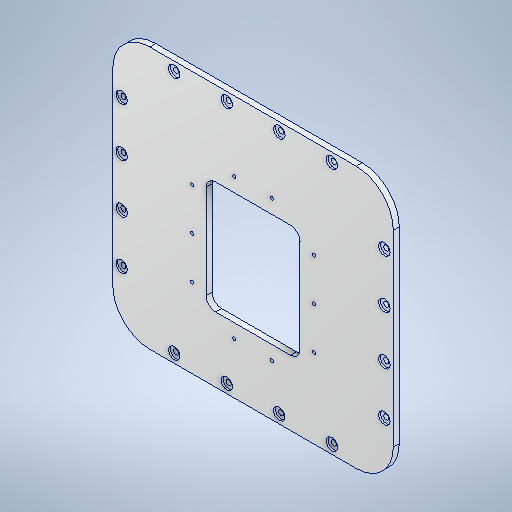
# Autodesk Inventor part: Reducer Plate
Saved by Autodesk Inventor 2025.2 (Build 292293000, 293)
## iProperties
Created: 2020-10-16
Part Number: Reducer Plate
Material: Aluminum 6061
Document SubType Name: Modeling
Designer: stabl
Density: 2.7 g/cm^3
Appearance: Aluminum - Flat
Author: stabl
Autodesk Inventor part; units mm, degrees
ref_plane "YZ Plane" through (0, 0, 0) normal (1, 0, 0) x (0, 1, 0)
ref_plane "XZ Plane" through (0, 0, 0) normal (0, 1, 0) x (-1, 0, 0)
ref_plane "Work Plane2" through (0, 0, 0) normal (0, 0, 1) x (1, 0, 0)
sketch "Sketch1" plane through (0, 0, 0) normal (0, 0, 1) x (1, 0, 0)
  line L0 (180, 126) -> (180, 200) projected
  arc A0 (180, 200) -> (175, 205) centre (175, 200) ccw projected
  line L1 (175, 205) -> (-174, 205) projected
  line L2 (-174, -368) -> (-174, 205) projected
  line L3 (-156, -368) -> (-174, -368) projected
  arc A1 (-153, -371) -> (-156, -368) centre (-156, -371) ccw projected
  line L4 (-153, -403) -> (-153, -371) projected
  arc A2 (-156, -406) -> (-153, -403) centre (-156, -403) ccw projected
  line L5 (-180, -406) -> (-156, -406) projected
  line L6 (-180, -406) -> (-180, -480) projected
  arc A3 (-180, -480) -> (-175, -485) centre (-175, -480) ccw projected
  line L7 (-175, -485) -> (174, -485) projected
  line L8 (174, 88) -> (174, -485) projected
  line L9 (156, 88) -> (174, 88) projected
  arc A4 (153, 91) -> (156, 88) centre (156, 91) ccw projected
  line L10 (153, 123) -> (153, 91) projected
  arc A5 (156, 126) -> (153, 123) centre (156, 123) ccw projected
  line L11 (180, 126) -> (156, 126) projected
  circle A6 centre (0, 0) radius 135 projected
  circle A7 centre (82.55, 185) radius 3 projected
  circle A8 centre (-82.55, 185) radius 3 projected
  circle A9 centre (82.55, -460) radius 3 projected
  circle A10 centre (-82.55, -460) radius 3 projected
  line L12 (-149.5, -195) -> (-149.5, -395)
  arc A11 (-149.5, -395) -> (-110, -434.5) centre (-110, -395) ccw
  line L13 (-110, -434.5) -> (110, -434.5)
  arc A12 (110, -434.5) -> (149.5, -395) centre (110, -395) ccw
  line L14 (149.5, -395) -> (149.5, -195)
  arc A13 (149.5, -195) -> (110, -155.5) centre (110, -195) ccw
  line L15 (110, -155.5) -> (-110, -155.5)
  arc A14 (-110, -155.5) -> (-149.5, -195) centre (-110, -195) ccw
  line L16 (40, -245) -> (-40, -245)
  line L17 (-50, -255) -> (-50, -355)
  line L18 (-40, -365) -> (40, -365)
  line L19 (50, -355) -> (50, -255)
  arc A15 (-40, -245) -> (-50, -255) centre (-40, -255) ccw
  arc A16 (50, -255) -> (40, -245) centre (40, -255) ccw
  arc A17 (40, -365) -> (50, -355) centre (40, -355) ccw
  arc A18 (-50, -355) -> (-40, -365) centre (-40, -355) ccw
  point P0 (115, -175)
  point P1 (-50, -365)
  point P2 (-50, -245)
  point P3 (50, -365)
  dimension "d1" = 100
  dimension "d2" = 120
  dimension "d3" = 10
  constraints: 16 end point, 16 point on circle, 8 centre point, 8 tangent, 6 point on line, 3 equal radius, 2 horizontal, 2 parallel, 1 perpendicular
  measures "d1" distance of point (50, -365) point (-50, -365)
  measures "d2" distance of point (-50, -365) point (-50, -245)
  measures "d3" radius of A15
extrude "Extrusion1" add sketch "Sketch1" along normal blind 6.35 contours A14 L15 A13 L14 A12 L13 A11 L12
sketch "Sketch2" plane through (0, 0, 6.35) normal (0, 0, 1) x (1, 0, 0)
  line L0 (180, 126) -> (180, 200) projected
  arc A0 (180, 200) -> (175, 205) centre (175, 200) ccw projected
  line L1 (175, 205) -> (-174, 205) projected
  line L2 (-174, -368) -> (-174, 205) projected
  line L3 (-156, -368) -> (-174, -368) projected
  arc A1 (-153, -371) -> (-156, -368) centre (-156, -371) ccw projected
  line L4 (-153, -403) -> (-153, -371) projected
  arc A2 (-156, -406) -> (-153, -403) centre (-156, -403) ccw projected
  line L5 (-180, -406) -> (-156, -406) projected
  line L6 (-180, -406) -> (-180, -480) projected
  arc A3 (-180, -480) -> (-175, -485) centre (-175, -480) ccw projected
  line L7 (-175, -485) -> (174, -485) projected
  line L8 (174, 88) -> (174, -485) projected
  line L9 (156, 88) -> (174, 88) projected
  arc A4 (153, 91) -> (156, 88) centre (156, 91) ccw projected
  line L10 (153, 123) -> (153, 91) projected
  arc A5 (156, 126) -> (153, 123) centre (156, 123) ccw projected
  line L11 (180, 126) -> (156, 126) projected
  circle A6 centre (0, 0) radius 135 projected
  circle A7 centre (-140, -217) radius 2 projected
  circle A8 centre (-140, -269) radius 2 projected
  circle A9 centre (-140, -321) radius 2 projected
  circle A10 centre (-140, -373) radius 2 projected
  circle A11 centre (-84, -425) radius 2 projected
  circle A12 centre (-28, -425) radius 2 projected
  circle A13 centre (28, -425) radius 2 projected
  circle A14 centre (84, -425) radius 2 projected
  circle A15 centre (140, -373) radius 2 projected
  circle A16 centre (140, -321) radius 2 projected
  circle A17 centre (140, -269) radius 2 projected
  circle A18 centre (140, -217) radius 2 projected
  circle A19 centre (84, -165) radius 2 projected
  circle A20 centre (28, -165) radius 2 projected
  circle A21 centre (-28, -165) radius 2 projected
  circle A22 centre (-84, -165) radius 2 projected
  line L12 (-130, -190) -> (-130, -400) projected
  arc A23 (-115, -175) -> (-130, -190) centre (-115, -190) ccw projected
  line L13 (115, -175) -> (-115, -175) projected
  arc A24 (130, -190) -> (115, -175) centre (115, -190) ccw projected
  line L14 (130, -400) -> (130, -190) projected
  arc A25 (115, -415) -> (130, -400) centre (115, -400) ccw projected
  line L15 (-115, -415) -> (115, -415) projected
  arc A26 (-130, -400) -> (-115, -415) centre (-115, -400) ccw projected
  circle A27 centre (82.55, 185) radius 3 projected
  circle A28 centre (-82.55, 185) radius 3 projected
  circle A29 centre (82.55, -460) radius 3 projected
  circle A30 centre (-82.55, -460) radius 3 projected
  constraints: 16 coincident
hole "Hole1" at (-140, -217, 6.35) at (-84, -165, 6.35) at (-28, -165, 6.35) at (28, -165, 6.35) at (84, -165, 6.35) at (-140, -269, 6.35) at (-140, -321, 6.35) at (-140, -373, 6.35) at (-84, -425, 6.35) at (-28, -425, 6.35) at (28, -425, 6.35) at (84, -425, 6.35) at (140, -373, 6.35) at (140, -321, 6.35) at (140, -269, 6.35) at (140, -217, 6.35) direction (0, 0, -1) diameter 5.5 end through all counterbore diameter 12.24 counterbore depth 2 clearance for "Hex Head Bolt" size "M5" standard "Ansi Metric M Profile"
sketch "Sketch3" plane through (0, 0, 6.35) normal (0, 0, 1) x (1, 0, 0)
  point P0 (0, 0)
  point P1 (-65, -305)
  point P2 (-65, -260)
  point P3 (-65, -350)
  point P4 (65, -305)
  point P5 (65, -260)
  point P6 (65, -350)
  point P7 (-20, -230)
  point P8 (20, -230)
  point P9 (-20, -380)
  point P10 (20, -380)
  dimension "d18" = 45
  dimension "d19" = 45
  dimension "d22" = 45
  dimension "d23" = 45
  measures "d18" distance of point (-65, -350) point (-65, -305)
  measures "d19" distance of point (-65, -305) point (-65, -260)
  measures "d22" distance of point (65, -305) point (65, -260)
  measures "d23" distance of point (65, -350) point (65, -305)
hole "Hole2" at (-65, -305, 6.35) at (-65, -260, 6.35) at (-65, -350, 6.35) at (65, -305, 6.35) at (65, -260, 6.35) at (65, -350, 6.35) at (-20, -230, 6.35) at (20, -230, 6.35) at (-20, -380, 6.35) at (20, -380, 6.35) direction (0, 0, -1) diameter 3.4587 depth 10.8 tip angle 118 thread size "M4x0.5" class "6H" standard "ANSI Metric M Profile"
body "Solid1"
